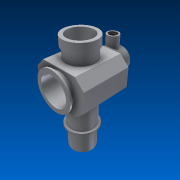
# Autodesk Inventor part: Carburetor Housing_v3
Saved by Autodesk Inventor 2016 (Build 200138000, 138)
## iProperties
Created: 2012-08-27
Part Number: Carburetor Housing_v3
Material: Aluminum 6061
Document SubType Name: Modeling
Designer: John
Density: 2.71 g/cm^3
Mass: 9.58727 g
Surface Area: 43.1099 cm^2
Volume: 3.53774 cm^3
Appearance: Aluminum - Flat
Author: John
Autodesk Inventor part; units mm, degrees
note: some values were not read from the file. Chosen so that the rebuilt part matches the saved one: direction of "Hole4".
ref_plane "YZ Plane" through (0, 0, 0) normal (1, 0, 0) x (0, 1, 0)
ref_plane "XZ Plane" through (0, 0, 0) normal (0, 1, 0) x (-1, 0, 0)
ref_plane "XY Plane" through (0, 0, 0) normal (0, 0, 1) x (1, 0, 0)
sketch "Sketch1" plane through (0, 0, 0) normal (0, 0, 1) x (1, 0, 0)
  line L0 (-9.6139, -8.7884) -> (9.6139, -8.7884)
  line L1 (9.6139, -8.7884) -> (9.6139, 8.7884)
  line L2 (9.6139, 8.7884) -> (-9.6139, 8.7884)
  line L3 (-9.6139, 8.7884) -> (-9.6139, -8.7884)
  line L4 (-9.6139, -8.7884) -> (9.6139, 8.7884) construction
  point P0 (0, 0)
  point P1 (0, 0)
  dimension "d0" = 19.2278
  dimension "d2" = 17.5768
  constraints: 10 end point, 2 parallel, 1 coincident, 1 horizontal, 1 midpoint, 1 perpendicular
  measures "d0" distance of L1.end L2.end
  measures "d2" distance of L0.end L1.end
extrude "Extrusion1" add sketch "Sketch1" along normal mid plane 13.1572
sketch "Sketch2" plane through (0, 0, 6.5786) normal (0, 0, 1) x (1, 0, 0)
  circle A0 centre (0, 0.6858) radius 5.3213
  line L0 (9.6139, 8.7884) -> (-9.6139, 8.7884) projected
  line L1 (-9.6139, -8.7884) -> (9.6139, -8.7884) projected
  line L2 (0, 8.7884) -> (0, -8.7884) construction
  dimension "d5" = 10.6426
  dimension "d9" = 8.1026
  constraints: 2 end point, 2 midpoint, 1 centre point, 1 point on line
  measures "d5" diameter of A0
  measures "d9" distance from line of L0 A0.centre
extrude "Extrusion2" add sketch "Sketch2" along normal blind 7.0612
sketch "Sketch3" plane through (0, 0, -6.5786) normal (0, 0, -1) x (-1, 0, 0)
  circle A0 centre (0, 0.6858) radius 5.3213 construction
  circle A1 centre (0, 0.6858) radius 5.3213
  dimension "d10" = 10.6426
  constraints: 1 centre point, 1 coincident
  measures "d10" diameter of A1
sketch "Sketch8" plane through (0, 0.6858, 13.6398) normal (0, 0, 1) x (1, 0, 0)
  circle A0 centre (0, 0) radius 5.3213 projected
  circle A1 centre (0, 0) radius 5.8674
  point P0 (0, -0.6858)
  dimension "d30" = 11.7348
  constraints: 1 centre point, 1 coincident
  measures "d30" diameter of A1
extrude "Extrusion3" add sketch "Sketch8" against normal blind 3.2512 contours A0 | A1
sketch "Sketch4" plane through (-9.6139, 8.7884, -6.5786) normal (0, 1, 0) x (1, 0, 0)
  line L0 (0, 0) -> (19.2278, -13.1572) construction
  circle A0 centre (9.6139, -6.5786) radius 5.715
  dimension "d13" = 11.43
  constraints: 2 end point, 1 centre point, 1 midpoint
  measures "d13" diameter of A0
extrude "Extrusion4" add sketch "Sketch3" along normal blind 10.2616
sketch "Sketch5" plane through (0, 11.0744, 0) normal (0, 1, 0) x (1, 0, 0)
  circle A0 centre (0, 0) radius 5.715 projected
  circle A1 centre (0, 0) radius 6.9596
  point P0 (0, 0)
  dimension "d17" = 13.9192
  constraints: 1 centre point, 1 coincident
  measures "d17" diameter of A1
sketch "Sketch12" plane through (0, 0.6858, -16.8402) normal (0, 0, -1) x (-1, 0, 0)
  circle A0 centre (0, 0) radius 5.3213 projected
  circle A1 centre (0, 0) radius 6.1595
  point P0 (0, -0.6858)
  dimension "d109" = 12.319
  constraints: 1 centre point, 1 coincident
  measures "d109" diameter of A1
extrude "Extrusion5" add sketch "Sketch12" along normal blind 0.8382 contours A0 | A1
sketch "Sketch13" plane through (0, 0.6858, -17.6784) normal (0, 0, -1) x (-1, 0, 0)
  circle A0 centre (0, 0) radius 6.1595 projected
  circle A1 centre (0, 0) radius 4.953
  dimension "d113" = 9.906
  constraints: 1 centre point, 1 coincident
  measures "d113" diameter of A1
extrude "Extrusion6" add sketch "Sketch13" along normal blind 8.763 contours A1
extrude "Extrusion7" add sketch "Sketch4" along normal blind 2.286
extrude "Extrusion8" add sketch "Sketch5" against normal blind 0.6858 contours A0 | A1
sketch "Sketch15" plane through (0, 0, 0) normal (1, 0, 0) x (0, 1, 0)
  line L0 (-16.9672, 0) -> (-16.9672, 4.1402)
  line L1 (6.0071, -6.5786) -> (6.0071, -16.8402) projected
  line L2 (-4.6355, -16.8402) -> (-4.6355, -6.5786) projected
  line L3 (-4.6355, -6.5786) -> (-8.7884, -6.5786) projected
  line L4 (-8.7884, -6.5786) -> (-8.7884, 6.5786) projected
  line L5 (-8.7884, 6.5786) -> (-4.6355, 6.5786) projected
  line L6 (-4.6355, 6.5786) -> (-4.6355, 10.3886) projected
  line L7 (-4.6355, 10.3886) -> (-5.1816, 10.3886) projected
  line L8 (-5.1816, 10.3886) -> (-5.1816, 13.6398) projected
  line L9 (-5.1816, 13.6398) -> (6.5532, 13.6398) projected
  line L10 (6.5532, 13.6398) -> (6.5532, 10.3886) projected
  line L11 (6.5532, 10.3886) -> (6.0071, 10.3886) projected
  line L12 (6.0071, 10.3886) -> (6.0071, 6.5786) projected
  line L13 (6.0071, 6.5786) -> (8.7884, 6.5786) projected
  line L14 (8.7884, 6.5786) -> (8.7884, 5.715) projected
  line L15 (8.7884, 5.715) -> (10.3886, 5.715) projected
  line L16 (10.3886, 5.715) -> (10.3886, 6.9596) projected
  line L17 (10.3886, 6.9596) -> (11.0744, 6.9596) projected
  line L18 (11.0744, 6.9596) -> (11.0744, -6.9596) projected
  line L19 (11.0744, -6.9596) -> (10.3886, -6.9596) projected
  line L20 (10.3886, -6.9596) -> (10.3886, -5.715) projected
  line L21 (10.3886, -5.715) -> (8.7884, -5.715) projected
  line L22 (8.7884, -5.715) -> (8.7884, -6.5786) projected
  line L23 (8.7884, -6.5786) -> (6.0071, -6.5786) projected
  line L24 (-8.7884, 0) -> (-16.9672, 0)
  line L25 (-16.9672, 4.1402) -> (-8.7884, 6.4008)
  line L26 (-8.7884, 0) -> (-8.7884, 6.4008)
  line L27 (6.0071, -16.8402) -> (6.8453, -16.8402) projected
  line L28 (6.8453, -16.8402) -> (6.8453, -17.6784) projected
  line L29 (6.8453, -17.6784) -> (5.6388, -17.6784) projected
  line L30 (5.6388, -17.6784) -> (5.6388, -26.4414) projected
  line L31 (5.6388, -26.4414) -> (-4.2672, -26.4414) projected
  line L32 (-4.2672, -26.4414) -> (-4.2672, -17.6784) projected
  line L33 (-4.2672, -17.6784) -> (-5.4737, -17.6784) projected
  line L34 (-5.4737, -17.6784) -> (-5.4737, -16.8402) projected
  line L35 (-5.4737, -16.8402) -> (-4.6355, -16.8402) projected
  point P0 (0, 0)
  dimension "d119" = 4.1402
  dimension "d136" = 8.1788
  dimension "d137" = 6.4008
  constraints: 8 end point, 1 collinear, 1 midpoint, 1 parallel, 1 point on line
  measures "d119" distance of L0.start L0.end
  measures "d136" distance of L24.start L0.start
  measures "d137" distance from line of L24 L25.end
revolve "Revolution1" add sketch "Sketch15" angle 360 about axis through (0, -8.7884, 0) along (0, -1, 0) contours L0 L25 L4 L24
sketch "Sketch17" plane through (0, 0, 0) normal (0, 0, 1) x (1, 0, 0)
  line L0 (-9.6139, -8.7884) -> (-9.6139, 8.7884) projected
  line L1 (-9.6139, 8.7884) -> (-5.715, 8.7884) projected
  line L2 (-5.715, 8.7884) -> (-5.715, 10.3886) projected
  line L3 (-5.715, 10.3886) -> (-6.9596, 10.3886) projected
  line L4 (-6.9596, 10.3886) -> (-6.9596, 11.0744) projected
  line L5 (-6.9596, 11.0744) -> (6.9596, 11.0744) projected
  line L6 (6.9596, 11.0744) -> (6.9596, 10.3886) projected
  line L7 (6.9596, 10.3886) -> (5.715, 10.3886) projected
  line L8 (5.715, 10.3886) -> (5.715, 8.7884) projected
  line L9 (5.715, 8.7884) -> (9.6139, 8.7884) projected
  line L10 (9.6139, 8.7884) -> (9.6139, -8.7884) projected
  line L11 (9.6139, -8.7884) -> (6.4008, -8.7884) projected
  line L12 (6.4008, -8.7884) -> (4.1402, -16.9672) projected
  line L13 (4.1402, -16.9672) -> (-4.1402, -16.9672) projected
  line L14 (-4.1402, -16.9672) -> (-6.4008, -8.7884) projected
  line L15 (-6.4008, -8.7884) -> (-9.6139, -8.7884) projected
  line L16 (0, -16.9672) -> (0, -12.7)
  circle A0 centre (0, -12.7) radius 2.2225
  point P0 (0, 0)
  dimension "d138" = 4.2672
  dimension "d139" = 4.445
  constraints: 2 end point, 1 centre point, 1 coincident, 1 midpoint, 1 perpendicular
  measures "d138" distance of L16.start L16.end
  measures "d139" diameter of A0
extrude "Extrusion9" add sketch "Sketch17" along normal blind 9.525 contours A0
hole "Hole1" at (0, 11.0744, 0) direction (0, -1, 0) diameter 10.5918 depth 16.8402
hole "Hole2" at (0, 0.6858, 13.6398) direction (0, 0, -1) diameter 9.0678 end through all
hole "Hole3" at (0, -16.9672, 0) direction (0, 1, 0) diameter 6.8072 end through all
hole "Hole4" at (0, -12.7, 9.525) direction (0, 0, -1) diameter 3.302 end up to surface thread size "8-32 UNC" class "2B" standard "ANSI Unified Screw Threads"
chamfer "Chamfer1" distance 3.175 angle 45 4 edges at (9.6139, 0, -6.5786) (-9.6139, 0, -6.5786) (9.6139, 0, 6.5786) (-9.6139, 0, 6.5786)
body "Solid1"
